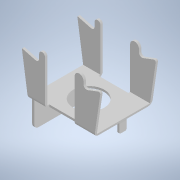
# Autodesk Inventor part: lock_washer_na
Saved by Autodesk Inventor 2021 (Build 250183000, 183)
## iProperties
Created: 2025-08-10
Part Number: lock_washer_na
Material: Generic
Catalog Web Link: www.cadenas.de
Description: LOCK WASHER-WALLMOUNT
Vendor: RITTAL
Document SubType Name: Modeling
Designer: psAdmin
Manufacturer: RITTAL
Mass: 0.633578 g
Surface Area: 19.3805 cm^2
Volume: 0.633578 cm^3
Density: 1 g/cm^3
Appearance: PSOLRGB-175-175-175
Category: PARTsolutions
Company: RITTAL
Title: lock_washer_na
Author: Cadenas PARTsolutions
Comments: WALLMOUNT
PSOL_IDENT_0: {$CADENAS_DATA/23d-libs/rittal/rittal_north_america/enclosure_systems/compact_enclosures/wm_parts/wm
PSOL_IDENT_1: _one_door_parts/lock_washer.prj},173 {VTYP=3D},{NB=lock_washer_na},{LINA=lock_washer_na},{NN=LOCK WA
PSOL_IDENT_2: SHER},{DATE=20.08.2024 09:24:21},{GEOMDATE=25.11.2019 11:27:18},{VERSION=},{LINEID=10},{WBVAR=},{WBN
PSOL_IDENT_3: UMERIC=}  {NB=lock_washer_na},{LINA=lock_washer_na},{KT=DUMMY},{PN=lock_washer},{DETAIL=MIN}
NB: lock_washer_na
NN: LOCK WASHER
NT: WALLMOUNT
NBSYN: $PN._na
LINA: lock_washer_na
CATALOG: Rittal
PN: lock_washer
DETAIL: 0
SUPPLIER: RITTAL
ARTICLENO: lock_washer_na
BOMINFO: lock_washer_na
CREATOR: CADENAS GmbH
Autodesk Inventor part; units mm, degrees
sketch "Sketch_1" plane through (0, 0, 0) normal (1, 0, 0) x (0, 1, 0)
  arc A0 (1.4, 9.75) -> (0, 8.35) centre (1.4, 8.35) ccw
  line L0 (0, 8.35) -> (0, -8.35)
  arc A1 (0, -8.35) -> (1.4, -9.75) centre (1.4, -8.35) ccw
  line L1 (1.4, -9.75) -> (16.2, -9.75)
  line L2 (16.2, -9.75) -> (16.2, -8.97)
  line L3 (16.2, -8.97) -> (0.7, -8.97)
  line L4 (0.7, -8.97) -> (0.7, 8.97)
  line L5 (0.7, 8.97) -> (16.2, 8.97)
  line L6 (16.2, 8.97) -> (16.2, 9.75)
  line L7 (16.2, 9.75) -> (1.4, 9.75)
  constraints: 16 end point, 4 point on circle, 2 centre point
extrude "Extrusion1" add sketch "Sketch_1" along normal mid plane 29.8667
sketch "Sketch_3" plane through (0, 0, 9.75) normal (0, 0, 1) x (1, 0, 0)
  line L0 (-22, 25) -> (-22, 0)
  line L1 (-22, 0) -> (-10.85, 0)
  line L2 (-10.85, 0) -> (-10.85, 0.7)
  line L3 (-10.85, 0.7) -> (-12.7818, 13.6261)
  arc A0 (-12.7301, 13.9322) -> (-12.7818, 13.6261) centre (-12.2873, 13.7) ccw
  line L4 (-12.7301, 13.9322) -> (-8.2588, 12.7341)
  arc A1 (-8.2588, 12.7341) -> (-7, 13.7) centre (-8, 13.7) ccw
  line L5 (-7, 13.7) -> (-7, 15.2)
  arc A2 (-5, 15.2) -> (-7, 15.2) centre (-6, 15.2) ccw
  line L6 (-5, 15.2) -> (-5, 0)
  line L7 (-5, 0) -> (5, 0)
  line L8 (5, 0) -> (5, 14.7)
  arc A3 (8, 14.7) -> (5, 14.7) centre (6.5, 14.7) ccw
  line L9 (8, 14.7) -> (8, 13.7)
  arc A4 (8, 13.7) -> (9.3545, 12.765) centre (9, 13.7) ccw
  line L10 (9.3545, 12.765) -> (13.1394, 14.2)
  arc A5 (13.6339, 13.6264) -> (13.1394, 14.2) centre (13.1394, 13.7) ccw
  line L11 (13.6339, 13.6264) -> (11.6047, 0)
  line L12 (11.6047, 0) -> (22, 0)
  line L13 (22, 0) -> (22, 25)
  line L14 (22, 25) -> (-22, 25)
  constraints: 30 end point, 12 point on circle, 6 centre point
extrude "Extrusion2" cut sketch "Sketch_3" against normal blind 1.4
sketch "Sketch_2" plane through (0, 0, -9.75) normal (0, 0, 1) x (1, 0, 0)
  line L0 (-22, 25) -> (-22, 0)
  line L1 (-22, 0) -> (-10.85, 0)
  line L2 (-10.85, 0) -> (-10.85, 0.7)
  line L3 (-10.85, 0.7) -> (-12.7818, 13.6261)
  arc A0 (-12.7301, 13.9322) -> (-12.7818, 13.6261) centre (-12.2873, 13.7) ccw
  line L4 (-12.7301, 13.9322) -> (-8.2588, 12.7341)
  arc A1 (-8.2588, 12.7341) -> (-7, 13.7) centre (-8, 13.7) ccw
  line L5 (-7, 13.7) -> (-7, 15.2)
  arc A2 (-5, 15.2) -> (-7, 15.2) centre (-6, 15.2) ccw
  line L6 (-5, 15.2) -> (-5, 0)
  line L7 (-5, 0) -> (5, 0)
  line L8 (5, 0) -> (5, 14.7)
  arc A3 (8, 14.7) -> (5, 14.7) centre (6.5, 14.7) ccw
  line L9 (8, 14.7) -> (8, 13.7)
  arc A4 (8, 13.7) -> (9.3545, 12.765) centre (9, 13.7) ccw
  line L10 (9.3545, 12.765) -> (13.1394, 14.2)
  arc A5 (13.6339, 13.6264) -> (13.1394, 14.2) centre (13.1394, 13.7) ccw
  line L11 (13.6339, 13.6264) -> (11.6047, 0)
  line L12 (11.6047, 0) -> (22, 0)
  line L13 (22, 0) -> (22, 25)
  line L14 (22, 25) -> (-22, 25)
  constraints: 30 end point, 12 point on circle, 6 centre point
extrude "Extrusion3" cut sketch "Sketch_2" along normal blind 1.4
sketch "Sketch4" plane through (-5, 0, 8.35) normal (0, -1, 0) x (1, 0, 0)
  point P0 (5, -8.35)
hole "Hole1" at (0, 0, 0) direction (0, 1, 0) diameter 10.5 depth 1
sketch "Sketch_5" plane through (0, 0, 0) normal (0, 0, 1) x (1, 0, 0)
  line L0 (-15.85, 1) -> (-15.85, -1)
  line L1 (-15.85, -1) -> (15.62, -1)
  line L2 (15.62, -1) -> (15.62, 1)
  line L3 (15.62, 1) -> (12.12, 1)
  line L4 (12.12, 1) -> (12.12, 0)
  line L5 (12.12, 0) -> (-10.85, 0)
  line L6 (-10.85, 0) -> (-10.85, 1)
  line L7 (-10.85, 1) -> (-15.85, 1)
  constraints: 16 end point
extrude "Extrusion4" cut sketch "Sketch_5" along normal mid plane 16.7
sketch "Sketch_9" plane through (0, 0, 9.75) normal (0, 0, 1) x (1, 0, 0)
  line L0 (11.6047, 0) -> (22, 0)
  line L1 (22, 0) -> (22, 25)
  line L2 (22, 25) -> (15.3276, 25)
  line L3 (15.3276, 25) -> (11.6047, 0)
  constraints: 8 end point
extrude "Extrusion5" cut sketch "Sketch_9" against normal blind 19.5
sketch "Sketch_6" plane through (-10.85, 0, 0) normal (1, 0, 0) x (0, 0, -1)
  arc A0 (-8.265, -7.8) -> (-6.765, -9.3) centre (-6.765, -7.8) ccw
  line L0 (-6.765, -9.3) -> (6.765, -9.3)
  arc A1 (6.765, -9.3) -> (8.265, -7.8) centre (6.765, -7.8) ccw
  line L1 (8.265, -7.8) -> (8.265, 0.7)
  line L2 (8.265, 0.7) -> (-8.265, 0.7)
  line L3 (-8.265, 0.7) -> (-8.265, -7.8)
  constraints: 8 end point, 4 point on circle, 2 centre point
extrude "Extrusion6" add sketch "Sketch_6" along normal blind 0.7
sketch "Sketch_7" plane through (0, 0, 0) normal (0, 0, 1) x (1, 0, 0)
  line L0 (10.8547, -3.3) -> (11.5547, -3.3)
  line L1 (11.5547, -3.3) -> (11.5547, -0.3252)
  line L2 (11.5547, -0.3252) -> (11.6047, 0)
  line L3 (11.6047, 0) -> (11.6047, 0.7)
  line L4 (11.6047, 0.7) -> (10.8547, 0.7)
  line L5 (10.8547, 0.7) -> (10.8547, -3.3)
  constraints: 12 end point
extrude "Extrusion7" add sketch "Sketch_7" along normal mid plane 2.5
sketch "Sketch_8" plane through (11.555, 0, 0) normal (1, 0, 0) x (0, 0, -1)
  line L0 (-1.5, -0.5) -> (-1.5, -4.5)
  line L1 (-1.5, -4.5) -> (1.5, -4.5)
  line L2 (1.5, -4.5) -> (1.5, -0.5)
  line L3 (1.5, -0.5) -> (1.25, -0.5)
  line L4 (1.25, -0.5) -> (1.25, -2.8)
  arc A0 (0.75, -3.3) -> (1.25, -2.8) centre (0.75, -2.8) ccw
  line L5 (0.75, -3.3) -> (-0.75, -3.3)
  arc A1 (-1.25, -2.8) -> (-0.75, -3.3) centre (-0.75, -2.8) ccw
  line L6 (-1.25, -2.8) -> (-1.25, -0.5)
  line L7 (-1.25, -0.5) -> (-1.5, -0.5)
  constraints: 16 end point, 4 point on circle, 2 centre point
extrude "Extrusion8" cut sketch "Sketch_8" against normal blind 0.78
ref_plane "washer_to_base_XY" through (0, -0.48, 0) normal (0, 1, 0) x (1, 0, 0)
ref_plane "washer_to_base_YZ" through (0, -0.48, 0) normal (1, 0, 0) x (0, 0, -1)
ref_plane "washer_to_base_ZX" through (0, -0.48, 0) normal (0, 0, -1) x (0, 1, 0)
ref_plane "washer_to_insert_XY" through (0, 0.7, 0) normal (0, 1, 0) x (1, 0, 0)
ref_plane "washer_to_insert_YZ" through (0, 0.7, 0) normal (1, 0, 0) x (0, 0, -1)
ref_plane "washer_to_insert_ZX" through (0, 0.7, 0) normal (0, 0, -1) x (0, 1, 0)
body "Solid1"
